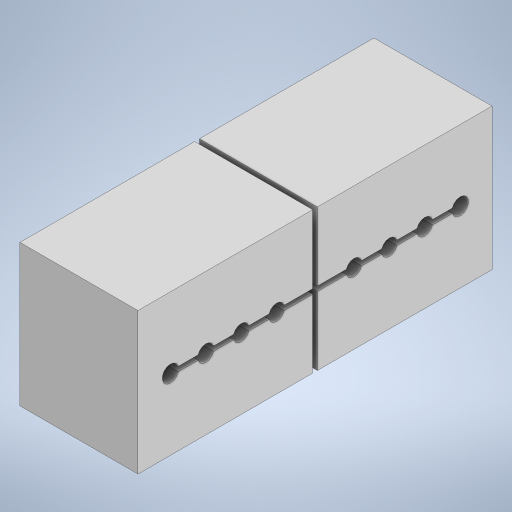
# Autodesk Inventor part: Prensa FOV2
Saved by Autodesk Inventor 2024.2 (Build 282272000, 272)
## iProperties
Created: 2025-08-06
Part Number: Prensa FOV2
Material: Generic
Document SubType Name: Modeling
Designer: ja.restrepo1
Density: 1 g/cm^3
Appearance: Default
Author: ja.restrepo1
Autodesk Inventor part; units mm, degrees
ref_plane "YZ Plane" through (0, 0, 0) normal (1, 0, 0) x (0, 1, 0)
ref_plane "XZ Plane" through (0, 0, 0) normal (0, 1, 0) x (-1, 0, 0)
ref_plane "XY Plane" through (0, 0, 0) normal (0, 0, 1) x (1, 0, 0)
sketch "Sketch1" plane through (0, 0, 0) normal (1, 0, 0) x (0, 1, 0)
  line L0 (6, 15) -> (-6, 15)
  line L1 (-6, 15) -> (-6, -15)
  line L2 (-6, -15) -> (6, -15)
  line L3 (6, -15) -> (6, 15)
  circle A0 centre (0, 12.25) radius 0.7
  line L4 (0.2, 15) -> (-0.2, 15)
  line L5 (-0.2, 15) -> (-0.2, -15)
  line L6 (-0.2, -15) -> (0.2, -15)
  line L7 (0.2, -15) -> (0.2, 15)
  line L8 (6, 0.2) -> (-6, 0.2)
  line L9 (-6, 0.2) -> (-6, -0.2)
  line L10 (-6, -0.2) -> (6, -0.2)
  line L11 (6, -0.2) -> (6, 0.2)
  circle A1 centre (0, 9.25) radius 0.69
  circle A2 centre (0, 6.25) radius 0.675
  circle A3 centre (0, 3.25) radius 0.675
  circle A4 centre (0, -3.3) radius 0.675
  circle A5 centre (0, -6.3) radius 0.675
  circle A6 centre (0, -9.3) radius 0.69
  circle A7 centre (0, -12.3) radius 0.7
  point P0 (0, 0)
  point P1 (6, 0)
  point P2 (0, 15)
  point P3 (0.2, 0)
  point P4 (0, 15)
  point P5 (-0.2, 11.5792)
  point P6 (-0.2, 12.9208)
  point P7 (0.2, 12.9208)
  point P8 (0.2, 11.5792)
  point P9 (-6, 0)
  point P10 (6, -0.2)
  point P11 (0.2, -0.2)
  point P12 (-0.2, -0.2)
  point P13 (-6, 0.2)
  point P14 (-0.2, 0.2)
  point P15 (0.2, 0.2)
  point P16 (-0.2, -11.6292)
  point P17 (-0.2, -9.9604)
  point P18 (-0.2, -8.6396)
  point P19 (-0.2, -6.9447)
  point P20 (-0.2, -5.6553)
  point P21 (-0.2, -3.9447)
  point P22 (-0.2, -2.6553)
  point P23 (0.2, -2.6553)
  point P24 (0.2, -3.9447)
  point P25 (0.2, -5.6553)
  point P26 (0.2, -6.9447)
  point P27 (0.2, -8.6396)
  point P28 (0.2, -9.9604)
  point P29 (0.2, -11.6292)
  point P30 (0.2, 3.8947)
  point P31 (0.2, 2.6053)
  point P32 (-0.2, 2.6053)
  point P33 (-0.2, 3.8947)
  point P34 (-0.2, 5.6053)
  point P35 (-0.2, 6.8947)
  point P36 (-0.2, 8.5896)
  point P37 (-0.2, 9.9104)
  point P38 (0.2, 9.9104)
  point P39 (0.2, 8.5896)
  point P40 (0.2, 6.8947)
  point P41 (0.2, 5.6053)
  dimension "d0" = 12
  dimension "d1" = 30
  dimension "d2" = 1.4
  dimension "d3" = 2.75
  dimension "d11" = 0.4
  dimension "d14" = 0.4
  dimension "d15" = 1.38
  dimension "d16" = 1.35
  dimension "d17" = 1.35
  dimension "d18" = 2.7
  dimension "d19" = 3
  dimension "d20" = 3
  dimension "d21" = 3
  dimension "d22" = 3
  dimension "d23" = 3
  dimension "d24" = 3
  constraints: 20 end point, 10 vertical alignment, 8 centre point, 5 parallel, 4 equal radius, 4 horizontal, 4 midpoint, 3 horizontal alignment, 2 collinear, 2 perpendicular, 1 point on line, 7 other
  measures "d0" distance of L0.start L0.end
  measures "d1" distance of L2.end L0.start
  measures "d2" diameter of A0
  measures "d3" distance from line of L0 A0.centre
  measures "d11" distance of L6.end L6.start
  measures "d14" distance between parallel lines of L8 L10
  measures "d15" diameter of A1
  measures "d16" diameter of A2
  measures "d17" diameter of A3
  measures "d18" distance from line of L2 A7.centre
  measures "d19" distance of A7.centre A6.centre
  measures "d20" distance of A6.centre A5.centre
  measures "d21" distance of A5.centre A4.centre
  measures "d22" distance of A3.centre A2.centre
  measures "d23" distance of A2.centre A1.centre
  measures "d24" distance of A1.centre A0.centre
extrude "Extrusion1" add sketch "Sketch1" along normal mid plane 10 contours L3 L8 L7 A3 A2 A1 A0 L0 | L7 A0 L5 L0 | L5 A0 A1 A2 A3 L8 L1 L0 | L3 L2 L7 A7 A6 A5 A4 L10 | L2 L5 A7 L7 | L5 A4 A5 A6 A7 L2 L1 L10
body "Solid1"
